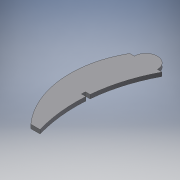
# Autodesk Inventor part: leg
Saved by Autodesk Inventor 2017 (Build 210142000, 142)
## iProperties
Created: 2018-12-03
Part Number: leg
Material: Generic
Document SubType Name: Modeling
Designer: Eric the Great
Density: 1 g/cm^3
Appearance: Default
Author: Eric the Great
Autodesk Inventor part; units mm, degrees
ref_plane "YZ Plane" through (0, 0, 0) normal (1, 0, 0) x (0, 1, 0)
ref_plane "XZ Plane" through (0, 0, 0) normal (0, 1, 0) x (-1, 0, 0)
ref_plane "XY Plane" through (0, 0, 0) normal (0, 0, 1) x (1, 0, 0)
sketch "Sketch1" plane through (0, 0, 0) normal (0, 0, 1) x (1, 0, 0)
  line L0 (-13.819, 82.4) -> (-7.5425, 82.4)
  line L1 (24.2075, 82.4) -> (30.484, 82.4)
  arc A0 (24.2075, 82.4) -> (-7.5425, 82.4) centre (8.3325, 82.4) ccw
  arc A1 (30.484, 82.4) -> (15.2091, -70) centre (209.6265, -12.5208) ccw
  line L2 (2.5091, -70) -> (15.2091, -70)
  arc A2 (-13.819, 82.4) -> (2.5091, -70) centre (99.9218, 17.5115) ccw
  point P0 (0, 0)
  dimension "d0" = 31.75
  dimension "d1" = 12.7
  dimension "d2" = 152.4
  dimension "d9" = 70
  constraints: 6 end point, 6 point on circle, 3 centre point, 2 horizontal, 2 horizontal alignment, 1 collinear, 1 line through centre
  measures "d0" distance of L1.start L0.end
  measures "d1" distance of L2.start L2.end
  measures "d2" distance between parallel lines of L2 L0
  measures "d9" distance from line of L2 point (0, 0)
extrude "Extrusion1" add sketch "Sketch1" along normal blind 5.3
sketch "Sketch2" plane through (0, 0, 5.3) normal (0, 0, 1) x (1, 0, 0)
  line L0 (1.2097, -6.5) -> (27.9202, -6.5)
  line L1 (27.9202, -6.5) -> (27.9202, -11.8)
  line L2 (27.9202, -11.8) -> (1.2097, -11.8)
  line L3 (1.2097, -11.8) -> (1.2097, -6.5)
  line L4 (-7.5425, 82.4) -> (-13.819, 82.4) projected
  point P0 (0, 0)
  dimension "d5" = 5.3
  dimension "d6" = 88.9
  constraints: 8 end point, 2 parallel, 1 horizontal, 1 perpendicular
  measures "d5" distance between parallel lines of L2 L0
  measures "d6" distance between parallel lines of L0 L4
extrude "Extrusion2" cut sketch "Sketch2" against normal up to surface (5.3 mm away)
body "Solid1"
